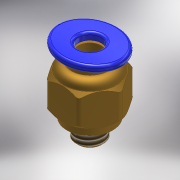
# Autodesk Inventor part: Clip pneumatique
Saved by Autodesk Inventor 2017 (Build 210142000, 142)
## iProperties
Company: FABLAB Frenchmakers
Part Number: Clip pneumatique
Material: ----------
Document SubType Name: Modeling
Designer: FABLAB Frenchmakers
Density: 7.86 g/cm^3
Appearance: Laiton - Satiné
Mass: 10.0649 g
Surface Area: 12.1809 cm^2
Volume: 1.28052 cm^3
Project: 1420 Vauban 3D XL
Catalog Web Link: http://frenchmakers.com/
Stock Number: 1420-05-19
Autodesk Inventor part; units mm, degrees
ref_plane "YZ Plane" through (0, 0, 0) normal (1, 0, 0) x (0, 1, 0)
ref_plane "XZ Plane" through (0, 0, 0) normal (0, 1, 0) x (-1, 0, 0)
sketch "Esquisse1" plane through (0, 0, 0) normal (0, 0, 1) x (1, 0, 0)
  line L0 (3.4641, 6) -> (6.9282, 0)
  line L1 (6.9282, 0) -> (3.4641, -6)
  line L2 (3.4641, -6) -> (-3.4641, -6)
  line L3 (-3.4641, -6) -> (-6.9282, 0)
  line L4 (-6.9282, 0) -> (-3.4641, 6)
  line L5 (-3.4641, 6) -> (3.4641, 6)
  point P0 (0, 0)
  point P1 (0, 0)
  dimension "d0" = 12
  constraints: 12 end point, 1 coincident, 1 horizontal, 13 other
  measures "d0" distance between parallel lines of L2 L5
extrude "Extrusion1" add sketch "Esquisse1" along normal mid plane 7
fillet "Congé2" radius 1 6 edges at (-6.9282, 0, 0) (-3.4641, -6, 0) (3.4641, -6, 0) (6.9282, 0, 0) (3.4641, 6, 0) (-3.4641, 6, 0)
sketch "Esquisse5" plane through (0, 0, 0) normal (0, 1, 0) x (-1, 0, 0)
  line L0 (-6.9282, 3.5) -> (-3.4641, 3.5) projected
  line L1 (-5.9282, 3.5) -> (-6.9282, 2.5)
  line L2 (-6.9282, 2.5) -> (-6.9282, -2.5)
  line L3 (-6.9282, -2.5) -> (-5.9282, -3.5)
  line L4 (-3.4641, -3.5) -> (-6.9282, -3.5) projected
  line L5 (-5.9282, -4.5) -> (-5.9282, -3.5)
  line L6 (-5.9282, -4.5) -> (-7.9282, -4.5)
  line L7 (-7.9282, -4.5) -> (-7.9282, 4.5)
  line L8 (-7.9282, 4.5) -> (-5.9282, 4.5)
  line L9 (-5.9282, 4.5) -> (-5.9282, 3.5)
  line L10 (-6.6395, 3.5) -> (-3.7528, 3.5) construction
  line L11 (-3.7528, -3.5) -> (-6.6395, -3.5) construction
  line L12 (0, -6.3) -> (0, 6.3) projected
  line L13 (-3.7528, 3.5) -> (-3.7528, -3.5) projected
  line L14 (-6.6395, -3.5) -> (-6.6395, 3.5) projected
  point P0 (0, 0)
  dimension "d13" = 45
  dimension "d14" = 1
  dimension "d15" = 1
  dimension "d16" = 1
  dimension "d17" = 1
  constraints: 16 end point, 7 perpendicular, 2 point on line, 1 horizontal
  measures "d13" angle of L0 L1
  measures "d14" distance between parallel lines of L0 L8
  measures "d15" distance between parallel lines of L4 L6
  measures "d16" distance between parallel lines of L7 L2
  measures "d17" horizontal distance of L1.start L1.end
revolve "Révolution1" cut sketch "Esquisse5" angle 360 about axis through (0, 0, -10) along (0, 0, 1) contours L14 L1 L2 L3 L4 L5 L6 L7 L8 L9 L0 | L0 L1 L14 | L3 L4 L14
sketch "Esquisse2" plane through (0, 0, -3.5) normal (0, 0, -1) x (-1, 0, 0)
  circle A0 centre (0, 0) radius 5
  dimension "d3" = 10
  constraints: 1 centre point, 1 coincident
  measures "d3" diameter of A0
extrude "Extrusion2" add sketch "Esquisse2" along normal blind 2
sketch "Esquisse3" plane through (0, 0, -5.5) normal (0, 0, -1) x (-1, 0, 0)
  circle A0 centre (0, 0) radius 3
  dimension "d6" = 6
  constraints: 1 centre point, 1 coincident
  measures "d6" diameter of A0
extrude "Extrusion3" add sketch "Esquisse3" along normal blind 4
chamfer "Chanfrein1" distance 0.5 angle 45 1 edges at (3, 0, -9.5)
sketch "Esquisse4" plane through (0, 0, 3.5) normal (0, 0, 1) x (1, 0, 0)
  circle A0 centre (0, 0) radius 5.825
  dimension "d9" = 11.65
  constraints: 1 centre point, 1 coincident
  measures "d9" diameter of A0
extrude "Extrusion4" add sketch "Esquisse4" along normal blind 1.75
fillet "Congé1" radius 1.75 1 edges at (-5.825, 0, 5.25)
sketch "Esquisse6" plane through (0, 0, 5.25) normal (0, 0, 1) x (1, 0, 0)
  circle A0 centre (0, 0) radius 4
  dimension "d20" = 8
  constraints: 1 centre point, 1 coincident
  measures "d20" diameter of A0
extrude "Extrusion5" add sketch "Esquisse6" along normal blind 1.5
thread "Filetage1" size "M6x1" class "6g" standard "ANSI Metric M Profile" full length
sketch "Esquisse7" plane through (0, 0, 6.75) normal (0, 0, 1) x (1, 0, 0)
  point P0 (0, 0)
  point P1 (0, 0)
  constraints: 1 coincident
hole "Perçage1" at (0, 0, 6.75) direction (0, 0, -1) diameter 3 end through all counterbore diameter 5 counterbore depth 11
ref_plane "Plan de construction1" through (0, 0, 7.25) normal (0, 0, 1) x (1, 0, 0)
sketch "Esquisse8" plane through (0, 0, 7.25) normal (0, 0, 1) x (1, 0, 0)
  circle A0 centre (0, 0) radius 1.5 projected
  ellipse E0 centre (0, 0) end of major axis (-7, 0) minor radius 6
  dimension "d33" = 6
  dimension "d34" = 7
  constraints: 1 coincident, 2 other
extrude "Extrusion6" add sketch "Esquisse8" along normal blind 1.5 separate body contours A0 | E0
sketch "Esquisse9" plane through (0, 0, 7.25) normal (0, 0, -1) x (-1, 0, 0)
  circle A0 centre (0, 0) radius 2.45
  dimension "d37" = 4.9
  constraints: 1 centre point, 1 coincident
  measures "d37" diameter of A0
extrude "Extrusion7" add sketch "Esquisse9" along normal blind 3 bodies 2
sketch "Esquisse10" plane through (0, 0, 8.75) normal (0, 0, 1) x (1, 0, 0)
  point P0 (0, 0)
  point P1 (0, 0)
  constraints: 1 coincident
hole "Perçage2" at (0, 0, 8.75) direction (0, 0, -1) diameter 5 end through all bodies 2
fillet "Congé3" radius 0.5 3 edges at (0, 2.5, 8.75) (7, 0, 8.75) (7, 0, 7.25)
equation "\"d15\" = d14"
equation "\"d12\" = d10"
equation "\"d10\" = 1.75"
